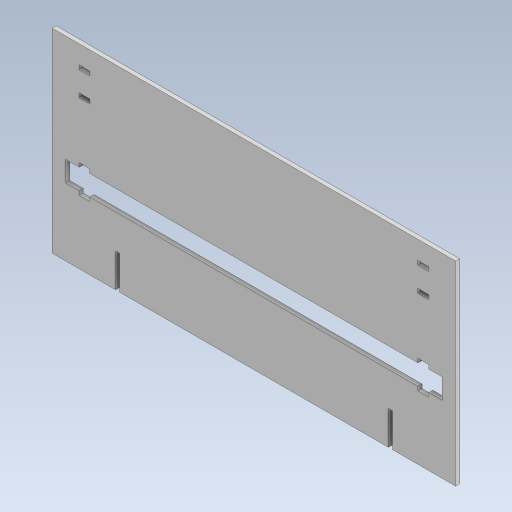
# Autodesk Inventor part: 零件5
Saved by Autodesk Inventor 2023 (Build 270158000, 158)
## iProperties
Created: 2023-05-12
Part Number: 零件5
Material: 一般
Document SubType Name: Modeling
Designer: Johnny Jou
Density: 1 g/cm^3
Appearance: 預設
Author: Johnny Jou
Autodesk Inventor part; units mm, degrees
ref_plane "YZ Plane" through (0, 0, 0) normal (1, 0, 0) x (0, 1, 0)
ref_plane "XZ Plane" through (0, 0, 0) normal (0, 1, 0) x (-1, 0, 0)
ref_plane "XY Plane" through (0, 0, 0) normal (0, 0, 1) x (1, 0, 0)
sketch "草圖1" plane through (0, 0, 0) normal (0, 0, 1) x (1, 0, 0)
  line L0 (0, 0) -> (300, 0)
  line L1 (300, 0) -> (300, -195)
  line L2 (300, -195) -> (0, -195)
  line L3 (0, -195) -> (0, 0)
  line L4 (20, -63.65) -> (28, -63.65)
  line L5 (28, -63.65) -> (28, -66.6)
  line L6 (28, -66.6) -> (20, -66.6)
  line L7 (20, -66.6) -> (20, -63.65)
  line L8 (20, -81.65) -> (28, -81.65)
  line L9 (28, -81.65) -> (28, -84.6)
  line L10 (28, -84.6) -> (20, -84.6)
  line L11 (20, -84.6) -> (20, -81.65)
  line L12 (20, -126.65) -> (28, -126.65)
  line L13 (28, -126.65) -> (28, -129.6)
  line L14 (28, -129.6) -> (20, -129.6)
  line L15 (20, -129.6) -> (20, -126.65)
  line L16 (20, -144.65) -> (28, -144.65)
  line L17 (28, -144.65) -> (28, -147.6)
  line L18 (28, -147.6) -> (20, -147.6)
  line L19 (20, -147.6) -> (20, -144.65)
  line L20 (280, -81.65) -> (280, -84.6)
  line L21 (280, -63.65) -> (280, -66.6)
  line L22 (272, -81.65) -> (280, -81.65)
  line L23 (280, -66.6) -> (272, -66.6)
  line L24 (272, -63.65) -> (280, -63.65)
  line L25 (280, -84.6) -> (272, -84.6)
  line L26 (272, -84.6) -> (272, -81.65)
  line L27 (272, -66.6) -> (272, -63.65)
  line L28 (272, -126.65) -> (280, -126.65)
  line L29 (280, -126.65) -> (280, -129.6)
  line L30 (272, -129.6) -> (272, -126.65)
  line L31 (280, -129.6) -> (272, -129.6)
  line L32 (272, -144.65) -> (280, -144.65)
  line L33 (280, -144.65) -> (280, -147.6)
  line L34 (280, -147.6) -> (272, -147.6)
  line L35 (272, -147.6) -> (272, -144.65)
  line L36 (0, -97.5) -> (300, -97.5) construction
  line L37 (24, -84.6) -> (24, -126.65) construction
  line L38 (150, 0) -> (150, -195) construction
  line L39 (28, -83.125) -> (272, -83.125) construction
  point P0 (20, -83.125)
  point P1 (20, -65.125)
  point P2 (20, -128.125)
  point P3 (20, -146.125)
  point P4 (272, -65.125)
  point P5 (272, -128.125)
  point P6 (272, -146.125)
  point P7 (150, -83.125)
  dimension "d0" = 2.95
  dimension "d1" = 8
  dimension "d2" = 18
  dimension "d3" = 45
  dimension "d4" = 18
  dimension "d5" = 195
  dimension "d6" = 300
  dimension "d9" = 252
  dimension "d16" = 12.9
  constraints: 80 end point, 12 midpoint, 11 point on line, 10 parallel, 6 horizontal, 6 perpendicular, 4 equal length, 36 other
  measures "d0" distance of L4.end L5.end
  measures "d1" distance of L4.start L4.end
  measures "d2" distance of point (20, -83.125) point (20, -65.125)
  measures "d3" distance of point (20, -128.125) point (20, -83.125)
  measures "d4" distance of point (20, -146.125) point (20, -128.125)
  measures "d5" distance of L0.end L1.end
  measures "d6" distance of L0.start L0.end
  measures "d9" distance of L5.end L21.end
  measures "d16" distance between parallel lines of L36 L10
extrude "擠出1" add sketch "草圖1" along normal blind 3
sketch "草圖3" plane through (0, 0, 3) normal (0, 0, 1) x (1, 0, 0)
  line L0 (300, 0) -> (0, 0) projected
  line L1 (0, 0) -> (300, 0)
  line L2 (300, 0) -> (300, -50)
  line L3 (300, -50) -> (0, -50)
  line L4 (0, -50) -> (0, 0)
  line L5 (300, -195) -> (300, 0) projected
  line L6 (47.05, -195) -> (50, -195)
  line L7 (50, -195) -> (50, -170)
  line L8 (50, -170) -> (47.05, -170)
  line L9 (47.05, -170) -> (47.05, -195)
  line L10 (0, -195) -> (300, -195) projected
  line L11 (250, -195) -> (252.95, -195)
  line L12 (252.95, -195) -> (252.95, -170)
  line L13 (252.95, -170) -> (250, -170)
  line L14 (250, -170) -> (250, -195)
  line L15 (50, -182.5) -> (250, -182.5)
  point P0 (150, -195)
  point P1 (150, -182.5)
  point P2 (252.95, -195)
  dimension "d17" = 50
  dimension "d18" = 200
  dimension "d19" = 2.95
  dimension "d20" = 2.95
  dimension "d21" = 25
  dimension "d22" = 25
  dimension "d23" = 0
  constraints: 26 end point, 6 parallel, 4 midpoint, 3 horizontal, 3 perpendicular, 2 collinear, 1 point on line
  measures "d17" distance of L1.end L2.end
  measures "d18" distance between parallel lines of L14 L7
  measures "d19" distance of L7.end L8.end
  measures "d20" distance of L12.end L13.end
  measures "d21" distance of L8.end L6.start
  measures "d22" distance of L11.end L12.end
  measures "d23" horizontal distance of point (150, -195) point (150, -182.5)
extrude "擠出2" cut sketch "草圖3" against normal up to surface (3 mm away) contours L2 L3 L4 L0 | L9 L8 L7 L6 | L14 L13 L12 L10
sketch "草圖6" plane through (0, 0, 3) normal (0, 0, 1) x (1, 0, 0)
  line L0 (290, -66.6) -> (290, -81.65) projected
  line L1 (10, -129.6) -> (290, -129.6)
  line L2 (290, -129.6) -> (290, -144.65)
  line L3 (290, -144.65) -> (10, -144.65)
  line L4 (10, -144.65) -> (10, -129.6)
  line L5 (28, -129.6) -> (20, -129.6) projected
  line L6 (20, -144.65) -> (28, -144.65) projected
  line L7 (0, -50) -> (0, -195) projected
  line L8 (300, -195) -> (300, -50) projected
  point P0 (0, 0)
  point P1 (290, -137.125)
  dimension "d32" = 10
  dimension "d33" = 10
  constraints: 8 end point, 2 collinear, 2 parallel, 1 horizontal, 1 midpoint, 1 perpendicular
  measures "d32" distance between parallel lines of L7 L4
  measures "d33" distance from line of L8 point (290, -137.125)
extrude "擠出5" cut sketch "草圖6" against normal up to surface (3 mm away)
